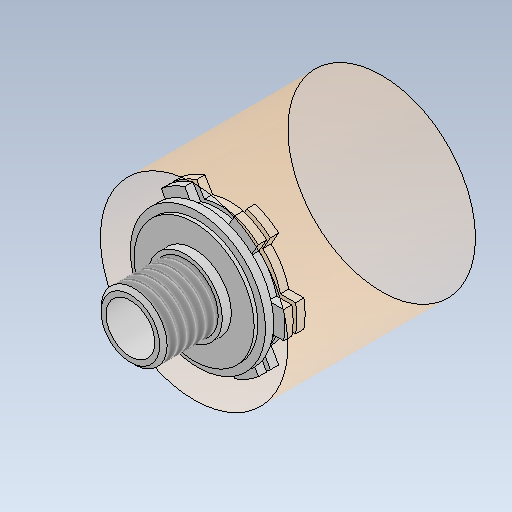
# Autodesk Inventor part: phon_jack
Saved by Autodesk Inventor 2026.1 (Build 301233020, 233B)
## iProperties
Created: 2026-08-13
Part Number: phon_jack
Material: 一般
Document SubType Name: Modeling
Designer: ug_nd
Density: 1 g/cm^3
Appearance: 既定
Author: ug_nd
Autodesk Inventor part; units mm, degrees
ref_plane "YZ Plane" through (0, 0, 0) normal (1, 0, 0) x (0, 1, 0)
ref_plane "XZ Plane" through (0, 0, 0) normal (0, 1, 0) x (-1, 0, 0)
ref_plane "XY Plane" through (0, 0, 0) normal (0, 0, 1) x (1, 0, 0)
sketch "スケッチ1" plane through (0, 0, 0) normal (0, 0, 1) x (1, 0, 0)
  circle A0 centre (0, 0) radius 8
  dimension "d0" = 16
  constraints: 1 centre point, 1 coincident
  measures "d0" diameter of A0
extrude "押し出し1" add sketch "スケッチ1" against normal blind 0.5
sketch "スケッチ2" plane through (0, 0, -0.5) normal (0, 0, -1) x (-1, 0, 0)
  circle A0 centre (0, 0) radius 9
  dimension "d3" = 18
  constraints: 1 centre point, 1 coincident
  measures "d3" diameter of A0
extrude "押し出し2" add sketch "スケッチ2" along normal blind 1.1
sketch "スケッチ3" plane through (0, 0, 0) normal (0, 0, 1) x (1, 0, 0)
  circle A0 centre (0, 0) radius 4.95
  dimension "d6" = 9.9
  constraints: 1 centre point, 1 coincident
  measures "d6" diameter of A0
extrude "押し出し3" add sketch "スケッチ3" along normal blind 1.2
sketch "スケッチ4" plane through (0, 0, -1.6) normal (0, 0, -1) x (-1, 0, 0)
  circle A0 centre (0, 0) radius 7
  dimension "d9" = 14
  constraints: 1 centre point, 1 coincident
  measures "d9" diameter of A0
extrude "押し出し4" add sketch "スケッチ4" along normal blind 0.5
sketch "スケッチ5" plane through (0, 0, -2.1) normal (0, 0, -1) x (-1, 0, 0)
  circle A0 centre (0, 0) radius 10 construction
  circle A1 centre (0, 0) radius 8 construction
  line L0 (-3.3595, 9.4188) -> (-2.3386, 7.6506)
  line L1 (0, -14) -> (0, 14) construction
  line L2 (14, 0) -> (-14, 0) construction
  arc A2 (2.3386, 7.6506) -> (-2.3386, 7.6506) centre (0, 0) ccw
  line L3 (3.3595, 9.4188) -> (2.3386, 7.6506)
  arc A3 (6.4772, 7.6188) -> (3.3595, 9.4188) centre (0, 0) ccw
  line L4 (-9.8367, 1.8) -> (-7.7949, 1.8)
  line L5 (-6.4772, 7.6188) -> (-5.4563, 5.8506)
  arc A4 (-3.3595, 9.4188) -> (-6.4772, 7.6188) centre (0, 0) ccw
  arc A5 (-5.4563, 5.8506) -> (-7.7949, 1.8) centre (0, 0) ccw
  line L6 (-6.4772, -7.6188) -> (-5.4563, -5.8506)
  line L7 (-9.8367, -1.8) -> (-7.7949, -1.8)
  arc A6 (-9.8367, 1.8) -> (-9.8367, -1.8) centre (0, 0) ccw
  arc A7 (-7.7949, -1.8) -> (-5.4563, -5.8506) centre (0, 0) ccw
  line L8 (3.3595, -9.4188) -> (2.3386, -7.6506)
  line L9 (-3.3595, -9.4188) -> (-2.3386, -7.6506)
  arc A8 (-6.4772, -7.6188) -> (-3.3595, -9.4188) centre (0, 0) ccw
  arc A9 (-2.3386, -7.6506) -> (2.3386, -7.6506) centre (0, 0) ccw
  line L10 (9.8367, -1.8) -> (7.7949, -1.8)
  line L11 (6.4772, -7.6188) -> (5.4563, -5.8506)
  arc A10 (3.3595, -9.4188) -> (6.4772, -7.6188) centre (0, 0) ccw
  arc A11 (5.4563, -5.8506) -> (7.7949, -1.8) centre (0, 0) ccw
  line L12 (6.4772, 7.6188) -> (5.4563, 5.8506)
  line L13 (9.8367, 1.8) -> (7.7949, 1.8)
  arc A12 (9.8367, -1.8) -> (9.8367, 1.8) centre (0, 0) ccw
  arc A13 (7.7949, 1.8) -> (5.4563, 5.8506) centre (0, 0) ccw
  dimension "d12" = 20
  dimension "d13" = 16
  dimension "d16" = 360
  dimension "d18" = 3.6
  constraints: 29 point on circle, 24 end point, 14 centre point, 4 coincident, 2 concentric, 2 symmetric about line, 1 parallel, 73 other
  measures "d12" diameter of A0
  measures "d13" diameter of A1
  measures "d18" distance between parallel lines of L5 L0
extrude "押し出し5" add sketch "スケッチ5" along normal blind 1.1
sketch "スケッチ6" plane through (0, 0, -3.2) normal (0, 0, -1) x (-1, 0, 0)
  circle A0 centre (0, 0) radius 7 projected
  circle A1 centre (0, 0) radius 7 projected
extrude "押し出し6" add sketch "スケッチ6" along normal blind 0.5
sketch "スケッチ7" plane through (0, 0, -3.7) normal (0, 0, -1) x (-1, 0, 0)
  circle A0 centre (0, 0) radius 7 construction
  arc A1 (-5.4563, 5.8506) -> (-7.7949, 1.8) centre (0, 0) ccw projected
  line L0 (-7.7949, 1.8) -> (-9.8367, 1.8) projected
  arc A2 (-9.8367, 1.8) -> (-9.8367, -1.8) centre (0, 0) ccw projected
  line L1 (-9.8367, -1.8) -> (-7.7949, -1.8) projected
  arc A3 (-7.7949, -1.8) -> (-5.4563, -5.8506) centre (0, 0) ccw projected
  line L2 (-5.4563, -5.8506) -> (-6.4772, -7.6188) projected
  arc A4 (-6.4772, -7.6188) -> (-3.3595, -9.4188) centre (0, 0) ccw projected
  line L3 (-3.3595, -9.4188) -> (-2.3386, -7.6506) projected
  arc A5 (-2.3386, -7.6506) -> (2.3386, -7.6506) centre (0, 0) ccw projected
  line L4 (2.3386, -7.6506) -> (3.3595, -9.4188) projected
  arc A6 (3.3595, -9.4188) -> (6.4772, -7.6188) centre (0, 0) ccw projected
  line L5 (6.4772, -7.6188) -> (5.4563, -5.8506) projected
  arc A7 (5.4563, -5.8506) -> (7.7949, -1.8) centre (0, 0) ccw projected
  line L6 (7.7949, -1.8) -> (9.8367, -1.8) projected
  arc A8 (9.8367, -1.8) -> (9.8367, 1.8) centre (0, 0) ccw projected
  line L7 (9.8367, 1.8) -> (7.7949, 1.8) projected
  arc A9 (7.7949, 1.8) -> (5.4563, 5.8506) centre (0, 0) ccw projected
  line L8 (5.4563, 5.8506) -> (6.4772, 7.6188) projected
  arc A10 (6.4772, 7.6188) -> (3.3595, 9.4188) centre (0, 0) ccw projected
  line L9 (3.3595, 9.4188) -> (2.3386, 7.6506) projected
  arc A11 (2.3386, 7.6506) -> (-2.3386, 7.6506) centre (0, 0) ccw projected
  line L10 (-2.3386, 7.6506) -> (-3.3595, 9.4188) projected
  arc A12 (-3.3595, 9.4188) -> (-6.4772, 7.6188) centre (0, 0) ccw projected
  line L11 (-6.4772, 7.6188) -> (-5.4563, 5.8506) projected
extrude "押し出し7" add sketch "スケッチ7" along normal blind 1.1
sketch "スケッチ8" plane through (0, 0, -4.8) normal (0, 0, -1) x (-1, 0, 0)
  circle A0 centre (0, 0) radius 6
  dimension "d25" = 12
  constraints: 1 centre point, 1 coincident
  measures "d25" diameter of A0
extrude "押し出し8" add sketch "スケッチ8" along normal blind 0.5
sketch "スケッチ9" plane through (0, 0, 1.2) normal (0, 0, 1) x (1, 0, 0)
  circle A0 centre (0, 0) radius 4.4
  dimension "d28" = 8.8
  constraints: 1 centre point, 1 coincident
  measures "d28" diameter of A0
extrude "押し出し9" add sketch "スケッチ9" along normal blind 7.3
thread "ねじ1" size "M9x1.25" class "6g" standard "ANSI Metric M Profile" full length
chamfer "面取り1" distance 0.5 angle 45 1 edges at (-4.4, 0, 8.5)
sketch "スケッチ10" plane through (0, 0, 8.5) normal (0, 0, 1) x (1, 0, 0)
  circle A0 centre (0, 0) radius 3.25
  dimension "d36" = 6.5
  constraints: 1 centre point, 1 coincident
  measures "d36" diameter of A0
extrude "押し出し10" cut sketch "スケッチ10" against normal through all
sketch "スケッチ11" plane through (0, 0, 0) normal (1, 0, 0) x (0, 1, 0)
  line L0 (0, -8.06) -> (0, 11.26) construction
  line L1 (-13.1863, 0) -> (13.1863, 0) construction
  line L2 (12.5, 0) -> (12.5, -25)
  point P0 (0, 0)
  dimension "d39" = 25
  dimension "d40" = 25
  constraints: 2 end point, 1 point on line, 1 vertical
  measures "d39" diameter of L2 L0
  measures "d40" distance of L2.start L2.end
surface revolve "回転サーフェス1" sketch "スケッチ11" angle 360 about axis through (0, 0, -10) along (0, 0, 1) shown yes curves L2
body "Srf1"
